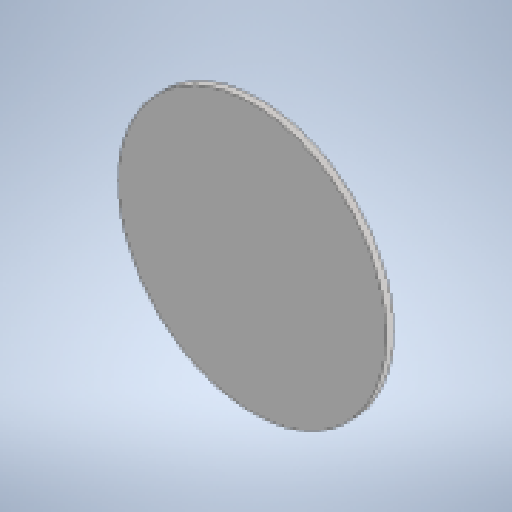
# Autodesk Inventor part: нижний эллипс головы
Saved by Autodesk Inventor 2023.1 (Build 271208000, 208)
## iProperties
Created: 2024-11-21
Part Number: нижний эллипс головы
Material: Типовые
Document SubType Name: Modeling
Designer: DELL
Density: 1 g/cm^3
Appearance: По умолчанию
Author: DELL
Autodesk Inventor part; units mm, degrees
ref_plane "YZ Plane" through (0, 0, 0) normal (1, 0, 0) x (0, 1, 0)
ref_plane "XZ Plane" through (0, 0, 0) normal (0, 1, 0) x (-1, 0, 0)
ref_plane "XY Plane" through (0, 0, 0) normal (0, 0, 1) x (1, 0, 0)
sketch "Эскиз1" plane through (0, 0, 0) normal (0, 0, 1) x (1, 0, 0)
  circle A0 centre (0, 0) radius 80
  line L0 (66, 54.4648) -> (48, 54.4648) projected
  line L1 (47, 52.4648) -> (47, 15.9648) projected
  line L2 (32, 54.4648) -> (51, 54.4648)
  line L3 (32, 15.9648) -> (32, 54.4648)
  line L4 (48, 13.9648) -> (66, 13.9648) projected
  line L5 (67, 15.9648) -> (67, 52.4648) projected
  line L6 (52, 54.4648) -> (32, 54.4648)
  line L7 (32, 54.4648) -> (32, 13.9648)
  line L8 (32, 13.9648) -> (52, 13.9648)
  line L9 (52, 13.9648) -> (52, 54.4648)
  point P0 (32, 52.4648)
  point P1 (52, 52.4648)
  point P2 (52, 15.9648)
  point P3 (52, 13.9648)
  point P4 (52, 54.4648)
  dimension "d2" = 160
  constraints: 12 end point, 2 horizontal, 2 parallel, 1 centre point, 1 perpendicular
  measures "d2" diameter of A0
extrude "Выдавливание1" add sketch "Эскиз1" against normal blind 4 contours A0 | L9 L4 L8 L7 L3 L2 L0
